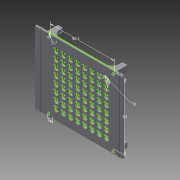
# Autodesk Inventor part: NUCholder
Saved by Autodesk Inventor 2015 (Build 190159000, 159)
## iProperties
Created: 2015-04-17
Part Number: NUCholder
Material: NylonD2W
Document SubType Name: Modeling
Designer: Akovo_000
Density: 0.93 g/cm^3
Appearance: Nylon 6
Mass: 27.2616 g
Surface Area: 250.408 cm^2
Volume: 29.3135 cm^3
Author: Akovo_000
Autodesk Inventor part; units mm, degrees
ref_plane "YZ Plane" through (0, 0, 0) normal (1, 0, 0) x (0, 1, 0)
ref_plane "XZ Plane" through (0, 0, 0) normal (0, 1, 0) x (-1, 0, 0)
ref_plane "XY Plane" through (0, 0, 0) normal (0, 0, 1) x (1, 0, 0)
sketch "NucSupport" plane through (0, 0, 0) normal (0, 1, 0) x (-1, 0, 0)
  line L0 (-28.8472, 8.4348) -> (-118.9472, 8.4348) construction
  line L1 (-118.9472, 8.4348) -> (-118.9472, 11.9348) construction
  line L2 (-118.9472, 101.4348) -> (-28.8472, 101.4348) construction
  line L3 (-28.8472, 101.4348) -> (-28.8472, 11.9348) construction
  line L4 (-143.4277, -0.0015) -> (-143.4277, -0.0016)
  line L5 (-25.3472, 4.9348) -> (-32.3472, 4.9348)
  line L6 (-32.3472, 4.9348) -> (-32.3472, 8.4348)
  line L7 (-32.3472, 11.9348) -> (-28.8472, 11.9348) construction
  line L8 (-25.3472, 11.9348) -> (-25.3472, 4.9348)
  line L9 (-25.3472, 4.9348) -> (-32.3472, 11.9348) construction
  line L10 (-32.3472, 4.9348) -> (-25.3472, 11.9348) construction
  line L11 (-25.3472, 97.9348) -> (-28.8472, 97.9348)
  line L12 (-32.3472, 97.9348) -> (-32.3472, 101.4348) construction
  line L13 (-32.3472, 104.9348) -> (-25.3472, 104.9348)
  line L14 (-25.3472, 104.9348) -> (-25.3472, 97.9348)
  line L15 (-25.3472, 97.9348) -> (-32.3472, 104.9348) construction
  line L16 (-32.3472, 97.9348) -> (-25.3472, 104.9348) construction
  line L17 (-115.4472, 97.9348) -> (-118.9472, 97.9348) construction
  line L18 (-122.4472, 97.9348) -> (-122.4472, 104.9348)
  line L19 (-122.4472, 104.9348) -> (-115.4472, 104.9348)
  line L20 (-115.4472, 104.9348) -> (-115.4472, 101.4348)
  line L21 (-115.4472, 97.9348) -> (-122.4472, 104.9348) construction
  line L22 (-122.4472, 97.9348) -> (-115.4472, 104.9348) construction
  line L23 (-115.4472, 4.9348) -> (-122.4472, 4.9348)
  line L24 (-122.4472, 4.9348) -> (-122.4472, 11.9348)
  line L25 (-122.4472, 11.9348) -> (-118.9472, 11.9348)
  line L26 (-115.4472, 11.9348) -> (-115.4472, 8.4348) construction
  line L27 (-115.4472, 4.9348) -> (-122.4472, 11.9348) construction
  line L28 (-122.4472, 4.9348) -> (-115.4472, 11.9348) construction
  arc A0 (-28.8472, 11.9348) -> (-32.3472, 8.4348) centre (-28.8472, 8.4348) ccw
  arc A1 (-32.3472, 101.4348) -> (-28.8472, 97.9348) centre (-28.8472, 101.4348) ccw
  line L29 (-118.9472, 11.9348) -> (-118.9472, 101.4348) construction
  line L30 (-32.3472, 8.4348) -> (-32.3472, 11.9348) construction
  line L31 (-28.8472, 11.9348) -> (-28.8472, 8.4348) construction
  line L32 (-28.8472, 97.9348) -> (-32.3472, 97.9348) construction
  line L33 (-32.3472, 101.4348) -> (-32.3472, 104.9348)
  line L34 (-115.4472, 101.4348) -> (-115.4472, 97.9348) construction
  line L35 (-118.9472, 97.9348) -> (-122.4472, 97.9348)
  line L36 (-28.8472, 11.9348) -> (-25.3472, 11.9348)
  line L37 (-115.4472, 8.4348) -> (-115.4472, 4.9348)
  line L38 (-118.9472, 11.9348) -> (-115.4472, 11.9348) construction
  arc A2 (-115.4472, 8.4348) -> (-118.9472, 11.9348) centre (-118.9472, 8.4348) ccw
  arc A3 (-118.9472, 97.9348) -> (-115.4472, 101.4348) centre (-118.9472, 101.4348) ccw
  circle A4 centre (-28.8472, 101.4348) radius 1.85
  circle A5 centre (-118.9472, 101.4348) radius 1.85
  circle A6 centre (-118.9472, 8.4348) radius 1.85
  circle A7 centre (-28.8472, 8.4348) radius 1.85
  line L39 (-25.3472, 4.9348) -> (-122.4472, 4.9348)
  line L40 (-122.4472, 4.9348) -> (-122.4472, 104.9348)
  line L41 (-122.4472, 104.9348) -> (-25.3472, 104.9348)
  line L42 (-25.3472, 104.9348) -> (-25.3472, 4.9348)
  circle A8 centre (-109.4101, 88.9977) radius 4
  circle A9 centre (-109.4101, 78.9977) radius 4
  circle A10 centre (-109.4101, 68.9977) radius 4
  circle A11 centre (-109.4101, 58.9977) radius 4
  circle A12 centre (-109.4101, 48.9977) radius 4
  circle A13 centre (-109.4101, 38.9977) radius 4
  circle A14 centre (-109.4101, 28.9977) radius 4
  circle A15 centre (-109.4101, 18.9977) radius 4
  circle A16 centre (-99.4101, 88.9977) radius 4
  circle A17 centre (-99.4101, 78.9977) radius 4
  circle A18 centre (-99.4101, 68.9977) radius 4
  circle A19 centre (-99.4101, 58.9977) radius 4
  circle A20 centre (-99.4101, 48.9977) radius 4
  circle A21 centre (-99.4101, 38.9977) radius 4
  circle A22 centre (-99.4101, 28.9977) radius 4
  circle A23 centre (-99.4101, 18.9977) radius 4
  circle A24 centre (-89.4101, 88.9977) radius 4
  circle A25 centre (-89.4101, 78.9977) radius 4
  circle A26 centre (-89.4101, 68.9977) radius 4
  circle A27 centre (-89.4101, 58.9977) radius 4
  circle A28 centre (-89.4101, 48.9977) radius 4
  circle A29 centre (-89.4101, 38.9977) radius 4
  circle A30 centre (-89.4101, 28.9977) radius 4
  circle A31 centre (-89.4101, 18.9977) radius 4
  circle A32 centre (-79.4101, 88.9977) radius 4
  circle A33 centre (-79.4101, 78.9977) radius 4
  circle A34 centre (-79.4101, 68.9977) radius 4
  circle A35 centre (-79.4101, 58.9977) radius 4
  circle A36 centre (-79.4101, 48.9977) radius 4
  circle A37 centre (-79.4101, 38.9977) radius 4
  circle A38 centre (-79.4101, 28.9977) radius 4
  circle A39 centre (-79.4101, 18.9977) radius 4
  circle A40 centre (-69.4101, 88.9977) radius 4
  circle A41 centre (-69.4101, 78.9977) radius 4
  circle A42 centre (-69.4101, 68.9977) radius 4
  circle A43 centre (-69.4101, 58.9977) radius 4
  circle A44 centre (-69.4101, 48.9977) radius 4
  circle A45 centre (-69.4101, 38.9977) radius 4
  circle A46 centre (-69.4101, 28.9977) radius 4
  circle A47 centre (-69.4101, 18.9977) radius 4
  circle A48 centre (-59.4101, 88.9977) radius 4
  circle A49 centre (-59.4101, 78.9977) radius 4
  circle A50 centre (-59.4101, 68.9977) radius 4
  circle A51 centre (-59.4101, 58.9977) radius 4
  circle A52 centre (-59.4101, 48.9977) radius 4
  circle A53 centre (-59.4101, 38.9977) radius 4
  circle A54 centre (-59.4101, 28.9977) radius 4
  circle A55 centre (-59.4101, 18.9977) radius 4
  circle A56 centre (-49.4101, 88.9977) radius 4
  circle A57 centre (-49.4101, 78.9977) radius 4
  circle A58 centre (-49.4101, 68.9977) radius 4
  circle A59 centre (-49.4101, 58.9977) radius 4
  circle A60 centre (-49.4101, 48.9977) radius 4
  circle A61 centre (-49.4101, 38.9977) radius 4
  circle A62 centre (-49.4101, 28.9977) radius 4
  circle A63 centre (-49.4101, 18.9977) radius 4
  circle A64 centre (-39.4101, 88.9977) radius 4
  circle A65 centre (-39.4101, 78.9977) radius 4
  circle A66 centre (-39.4101, 68.9977) radius 4
  circle A67 centre (-39.4101, 58.9977) radius 4
  circle A68 centre (-39.4101, 48.9977) radius 4
  circle A69 centre (-39.4101, 38.9977) radius 4
  circle A70 centre (-39.4101, 28.9977) radius 4
  circle A71 centre (-39.4101, 18.9977) radius 4
  dimension "d73" = 90.1
  dimension "d74" = 93
  dimension "d281" = 7
  dimension "d284" = 3.7
  dimension "d295" = 8
  dimension "d298" = 10
  dimension "d301" = 10
  constraints: 86 end point, 72 centre point, 19 parallel, 12 perpendicular, 8 horizontal, 8 midpoint, 8 point on circle, 8 tangent, 7 coincident, 6 equal radius, 3 point on line, 2 vertical, 126 other
  measures "d73" distance of L2.start L2.end
  measures "d74" distance of L0.end L2.start
  measures "d281" distance of L5.start L5.end
  measures "d284" diameter of A4
  measures "d295" diameter of A8
  measures "d298" distance of A8.centre A9.centre
  measures "d301" distance of A8.centre A16.centre
extrude "NucAttachments" add sketch "NucSupport" along normal blind 14.5 contours L5 L6 A0 L36 L8 | L23 L24 L25 A2 L37 | L11 A1 L33 L13 L14 | L18 L19 L20 A3 L35
extrude "PLateForMaterial" add sketch "NucSupport" against normal blind 2.5
sketch "Sketch14" plane through (0, -2.5, 0) normal (0, -1, 0) x (1, 0, 0)
  circle A0 centre (28.8472, 8.4348) radius 1.85 projected
  line L0 (31.5472, 6.8759) -> (28.8472, 5.3171)
  line L1 (28.8472, 5.3171) -> (26.1472, 6.8759)
  line L2 (26.1472, 6.8759) -> (26.1472, 9.9936)
  line L3 (26.1472, 9.9936) -> (28.8472, 11.5525)
  line L4 (28.8472, 11.5525) -> (31.5472, 9.9936)
  line L5 (31.5472, 9.9936) -> (31.5472, 6.8759)
  circle A1 centre (28.8472, 101.4348) radius 1.85 projected
  line L6 (31.5472, 102.9936) -> (31.5472, 99.8759)
  line L7 (31.5472, 99.8759) -> (28.8472, 98.3171)
  line L8 (28.8472, 98.3171) -> (26.1472, 99.8759)
  line L9 (26.1472, 99.8759) -> (26.1472, 102.9936)
  line L10 (26.1472, 102.9936) -> (28.8472, 104.5525)
  line L11 (28.8472, 104.5525) -> (31.5472, 102.9936)
  circle A2 centre (118.9472, 101.4348) radius 1.85 projected
  line L12 (116.2472, 102.9936) -> (118.9472, 104.5525)
  line L13 (118.9472, 104.5525) -> (121.6472, 102.9936)
  line L14 (121.6472, 102.9936) -> (121.6472, 99.8759)
  line L15 (121.6472, 99.8759) -> (118.9472, 98.3171)
  line L16 (118.9472, 98.3171) -> (116.2472, 99.8759)
  line L17 (116.2472, 99.8759) -> (116.2472, 102.9936)
  circle A3 centre (118.9472, 8.4348) radius 1.85 projected
  line L18 (25.3472, 104.9348) -> (25.3472, 4.9348) projected
  line L19 (121.6472, 9.9936) -> (121.6472, 6.8759)
  line L20 (121.6472, 6.8759) -> (118.9472, 5.3171)
  line L21 (118.9472, 5.3171) -> (116.2472, 6.8759)
  line L22 (116.2472, 6.8759) -> (116.2472, 9.9936)
  line L23 (116.2472, 9.9936) -> (118.9472, 11.5525)
  line L24 (118.9472, 11.5525) -> (121.6472, 9.9936)
  arc A4 (35.3472, 4.9348) -> (25.3472, 14.9348) centre (25.3472, 4.9348) ccw
  line L25 (122.4472, 97.9348) -> (122.4472, 11.9348) projected
  arc A5 (122.4472, 14.9348) -> (112.4472, 4.9348) centre (122.4472, 4.9348) ccw
  arc A6 (112.4472, 104.9348) -> (122.4472, 94.9348) centre (122.4472, 104.9348) ccw
  line L26 (32.3472, 104.9348) -> (115.4472, 104.9348) projected
  arc A7 (25.3472, 94.9348) -> (35.3472, 104.9348) centre (25.3472, 104.9348) ccw
  line L27 (112.4472, 4.9348) -> (122.4472, 4.9348)
  line L28 (25.3472, 4.9348) -> (122.4472, 4.9348) projected
  line L29 (122.4472, 4.9348) -> (122.4472, 14.9348)
  line L30 (112.4472, 104.9348) -> (122.4472, 104.9348)
  line L31 (122.4472, 104.9348) -> (122.4472, 94.9348)
  line L32 (35.3472, 104.9348) -> (25.3472, 104.9348)
  line L33 (25.3472, 104.9348) -> (25.3472, 94.9348)
  line L34 (35.3472, 4.9348) -> (25.3472, 4.9348)
  line L35 (25.3472, 4.9348) -> (25.3472, 14.9348)
  line L36 (25.3472, 11.9348) -> (25.3472, 97.9348) projected
  point P0 (0, 0)
  dimension "d291" = 5.4
  dimension "d292" = 10
  constraints: 64 end point, 8 point on circle, 7 coincident, 7 collinear, 4 centre point, 4 point on line, 3 equal length, 3 equal radius, 2 horizontal, 2 parallel, 1 perpendicular, 52 other
  measures "d291" distance between parallel lines of L0 L3
  measures "d292" radius of A4
extrude "Extrusion18" cut sketch "Sketch14" against normal blind 2.5 contours L0 L1 L2 L3 L4 L5 | L6 L7 L8 L9 L10 L11 | L12 L13 L14 L15 L16 L17 | L19 L20 L21 L22 L23 L24
fillet "Fillet1" radius 10 12 edges at (116.4723, 0, 98.9599) (115.4472, 0, 103.1848) (120.6972, 0, 97.9348) (32.3472, 0, 103.1848) (27.0972, 0, 97.9348) (31.3221, 0, 98.9599) (27.0972, 0, 11.9348) (32.3472, 0, 6.6848) (31.3221, 0, 10.9096) (116.4723, 0, 10.9096) (115.4472, 0, 6.6848) (120.6972, 0, 11.9348)
sketch "Sketch17" plane through (115.4472, 14.5, 104.9348) normal (0, 0, 1) x (1, 0, 0)
  line L0 (7, -17) -> (17, -17)
  line L1 (17, -17) -> (17, -14.5)
  line L2 (17, -14.5) -> (7, -14.5)
  line L3 (7, -14.5) -> (7, -17)
  line L4 (-90.1, -17) -> (-105.1, -17)
  line L5 (-105.1, -17) -> (-105.1, -14.5)
  line L6 (-105.1, -14.5) -> (-90.1, -14.5)
  line L7 (-90.1, -14.5) -> (-90.1, -17)
  line L8 (12, -17) -> (12, -16.65)
  line L9 (-97.6, -17) -> (-97.6, -16.65)
  circle A0 centre (12, -15.75) radius 0.9
  circle A1 centre (-97.6, -15.75) radius 0.9
  circle A2 centre (12, -15.75) radius 2
  circle A3 centre (-97.6, -15.75) radius 2
  line L10 (-97.6, -14.85) -> (-97.6, -14.5)
  line L11 (-97.6, -15.75) -> (-97.6, -16.65) construction
  line L12 (-97.6, -15.75) -> (-97.6, -14.85) construction
  line L13 (12, -14.85) -> (12, -14.5)
  line L14 (12, -15.75) -> (12, -16.65) construction
  line L15 (12, -15.75) -> (12, -14.85) construction
  point P0 (-115.4472, -14.5)
  dimension "d312" = 10
  dimension "d313" = 15
  dimension "d315" = 1.8
  dimension "d316" = 2.5
  dimension "d317" = 4
  constraints: 32 end point, 6 equal length, 4 centre point, 4 midpoint, 4 point on circle, 3 collinear, 2 coincident, 2 equal radius, 2 horizontal, 2 perpendicular, 2 vertical, 1 point on line
  measures "d312" distance of L2.end L1.end
  measures "d313" distance of L5.end L6.end
  measures "d315" diameter of A1
  measures "d316" distance between parallel lines of L0 L2
  measures "d317" diameter of A2
extrude "Extrusion20" add sketch "Sketch17" against normal blind 100 contours L3 L2 A2 L0 | A2 L2 L13 A0 L8 L0 | L0 A2 | L8 A0 L13 L2 A2 L0 | A2 L2 | A2 L2 L1 L0 | L4 A3 L6 L7 | A3 L4 | L4 L9 A1 L10 L6 A3 | L4 A3 L6 L10 A1 L9 | L4 L5 L6 A3 | L6 A3
body "Solid3"
